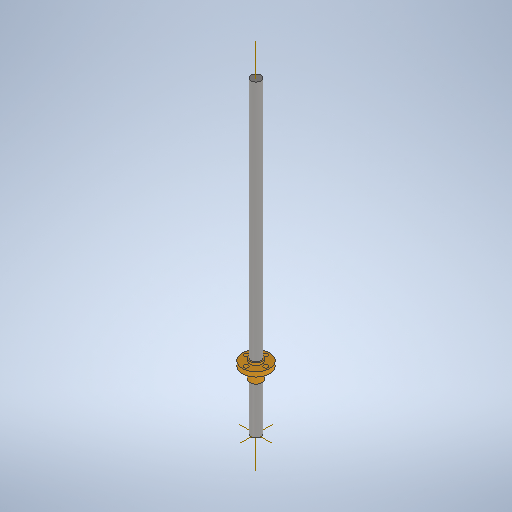
# Autodesk Inventor part: Lead screw
Saved by Autodesk Inventor 2025.2 (Build 292293000, 293)
## iProperties
Created: 2025-01-25
Part Number: Lead screw
Material: Generic
Document SubType Name: Modeling
Designer: caomi
Density: 1 g/cm^3
Appearance: Default
Author: caomi
Autodesk Inventor part; units mm, degrees
ref_plane "YZ Plane" through (0, 0, 0) normal (1, 0, 0) x (0, 1, 0)
ref_plane "XZ Plane" through (0, 0, 0) normal (0, 1, 0) x (-1, 0, 0)
ref_plane "XY Plane" through (0, 0, 0) normal (0, 0, 1) x (1, 0, 0)
sketch "Sketch1" plane through (0, 0, 0) normal (0, 1, 0) x (-1, 0, 0)
  circle A0 centre (0, 0) radius 4
  dimension "d6" = 8
  constraints: 1 centre point, 1 coincident
  measures "d6" diameter of A0
extrude "Extrusion1" add sketch "Sketch1" along normal blind 250
sketch "Sketch3" plane through (0, 0, 0) normal (0, 0, 1) x (1, 0, 0)
  line L0 (3.9002, 53.4648) -> (3.9002, 38.4648)
  line L1 (3.9002, 38.4648) -> (4.9, 38.4648)
  line L2 (4.9, 38.4648) -> (4.9, 47.7648)
  line L3 (4.9, 47.7648) -> (11, 47.7648)
  line L4 (11, 47.7648) -> (11, 51.4648)
  line L5 (0, -50) -> (0, 300) projected
  line L6 (11, 51.4648) -> (4.9, 51.4648)
  line L7 (4.9, 51.4648) -> (4.9, 53.4648)
  line L8 (4.9, 53.4648) -> (3.9002, 53.4648)
  point P0 (0, 0)
  point P1 (11, 49.6148)
  point P2 (4.4001, 38.4648)
  dimension "d10" = 11
  dimension "d11" = 6.1
  dimension "d13" = 2
  dimension "d14" = 15
  dimension "d15" = 3.7
  constraints: 16 end point, 6 perpendicular, 2 midpoint, 1 collinear, 1 horizontal, 1 vertical
  measures "d10" distance from line of point (11, 49.615) L5
  measures "d11" distance of L2.end L3.end
  measures "d13" distance of L6.end L7.end
  measures "d14" distance from line of L8 point (4.4, 38.465)
  measures "d15" distance of L3.end L4.end
revolve "Revolution1" add sketch "Sketch3" angle 360 about axis through (0, -10, 0) along (0, 1, 0) separate body
sketch "Sketch4" plane through (0, 51.4648, 0) normal (0, 1, 0) x (1, 0, 0)
  circle A0 centre (-8, 0) radius 1.75
  point P0 (0, 0)
  dimension "d16" = 3.5
  dimension "d17" = 8
  constraints: 1 centre point
  measures "d16" diameter of A0
  measures "d17" distance of A0.centre point (0, 0)
extrude "Extrusion2" cut sketch "Sketch4" against normal blind 250 bodies 2
pattern_circular "Circular Pattern1" count 4 over 360 about axis through (0, 49.6148, 0) along (0, 1, 0) of "Extrusion2" bodies 2
body "Solid1"
body "Solid2"
